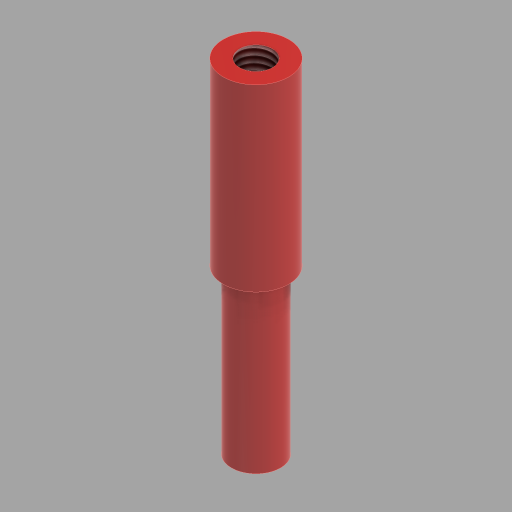
# Autodesk Inventor part: Fitting-2
Saved by Autodesk Inventor 2024 (Build 280153020, 153B)
## iProperties
Created: 2023-09-24
Part Number: Fitting-2
Material: Brass
Document SubType Name: Modeling
Designer: schanen
Density: 8.49 g/cm^3
Appearance: Orange-Red
Author: schanen
Autodesk Inventor part; units mm, degrees
ref_plane "YZ Plane" through (0, 0, 0) normal (1, 0, 0) x (0, 1, 0)
ref_plane "XZ Plane" through (0, 0, 0) normal (0, 1, 0) x (-1, 0, 0)
ref_plane "XY Plane" through (0, 0, 0) normal (0, 0, 1) x (1, 0, 0)
sketch "Sketch1" plane through (0, 0, 0) normal (0, 0, 1) x (1, 0, 0)
  line L0 (0, 11) -> (-1, 11)
  line L1 (-1, 11) -> (-1, 21)
  line L2 (-1, 21) -> (-2, 21)
  line L3 (-2, 21) -> (-2, 10)
  line L4 (-2, 10) -> (-1.5, 10)
  line L5 (-1.5, 10) -> (-1.5, 0)
  line L6 (-1.5, 0) -> (0, 0)
  line L7 (0, 0) -> (0, 11)
  dimension "d0" = 1
  dimension "d1" = 1.5
  dimension "d3" = 10
  dimension "d5" = 11
  dimension "d9" = 10
  dimension "d12" = 1
  constraints: 16 end point, 6 perpendicular, 1 coincident, 1 horizontal, 1 vertical, 1 vertical alignment
  measures "d0" distance between parallel lines of L7 L1
  measures "d1" distance between parallel lines of L7 L5
  measures "d3" distance of L4.end L5.end
  measures "d5" distance of L2.end L3.end
  measures "d9" distance of L0.end L1.end
  measures "d12" distance between parallel lines of L3 L1
revolve "Revolution1" add sketch "Sketch1" angle 360 about axis through (0, 0, 0) along (0, 1, 0)
thread "Thread4" size "M2x0.4" class "6H" standard "ANSI Metric M Profile" full length
body "Solid1"
